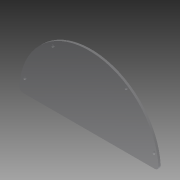
# Autodesk Inventor part: Top Plate
Saved by Autodesk Inventor 2015 (Build 190159000, 159)
## iProperties
Created: 2016-09-20
Part Number: Top Plate
Material: Generic
Document SubType Name: Modeling
Designer: James Yelland
Density: 1 g/cm^3
Appearance: Default
Author: James Yelland
Autodesk Inventor part; units mm, degrees
ref_plane "YZ Plane" through (0, 0, 0) normal (1, 0, 0) x (0, 1, 0)
ref_plane "XZ Plane" through (0, 0, 0) normal (0, 1, 0) x (-1, 0, 0)
ref_plane "XY Plane" through (0, 0, 0) normal (0, 0, 1) x (1, 0, 0)
sketch "Sketch1" plane through (0, 0, 0) normal (0, 1, 0) x (-1, 0, 0)
  circle A0 centre (50.0013, 74.8323) radius 1.6
  circle A1 centre (-50.0013, 74.8323) radius 1.6
  circle A2 centre (-88.2707, 17.5581) radius 1.6
  circle A3 centre (88.2707, 17.5581) radius 1.6
  line L0 (0, 0) -> (89.861, 0)
  line L1 (0, 0) -> (-89.861, 0)
  arc A4 (94.8533, 5.2778) -> (-94.8533, 5.2778) centre (0, 0) ccw
  arc A5 (89.861, 0) -> (94.8533, 5.2778) centre (89.861, 5) ccw
  arc A6 (-94.8533, 5.2778) -> (-89.861, 0) centre (-89.861, 5) ccw
  point P0 (95, 0)
  point P1 (-95, 0)
  dimension "d39" = 3.2
  dimension "d40" = 3.2
  dimension "d41" = 3.2
  dimension "d43" = 5
  constraints: 8 point on circle, 7 centre point, 4 end point, 4 tangent, 2 horizontal, 2 point on line, 1 coincident, 1 equal radius
  measures "d39" diameter of A1
  measures "d40" diameter of A2
  measures "d41" diameter of A3
  measures "d43" radius of A5
extrude "Extrusion1" add sketch "Sketch1" along normal blind 3
body "Solid1"
